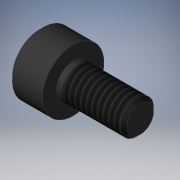
# Autodesk Inventor part: E-GSCB3-6
Saved by Autodesk Inventor 2019 (Build 230136000, 136)
## iProperties
Created: 2024-02-19
Part Number: E-GSCB3-6
Material: Generic
Catalog Web Link: www.cadenas.de
Description: E-GSCB-Economy Hexagon Socket Head Cap Screws - Stainless Steel
Vendor: MISUMI
Document SubType Name: Modeling
Designer: psAdmin
Manufacturer: MISUMI
Mass: 0.103858 g
Surface Area: 1.64097 cm^2
Volume: 0.103858 cm^3
Density: 1 g/cm^3
Appearance: PSOLRGB-175-175-175
Category: PARTsolutions
Company: MISUMI
Title: E-GSCB3-6
Author: Cadenas PARTsolutions
Comments: Economy Hexagon Socket Head Cap Screws - Stainless Steel
PSOL_IDENT_0: {$CADENAS_DATA/23d-libs/misumi/metric/27_screws_nuts/e_gscb.prj},160 {VTYP=3D},{NB=E-GSCB3-6},{LINA=
PSOL_IDENT_1: E-GSCB3-6},{NN=E-GSCB},{DATE=20.09.2023 07:17:35},{GEOMDATE=14.09.2023 02:41:30},{VERSION=},{LINEID=
PSOL_IDENT_2: 60},{WBVAR=L},{WBNUMERIC=L}  {NB=E-GSCB3-6},{LINA=E-GSCB3-6},{KT=DUMMY},{PN=E-GSCB3-6},{TYPE=E-GSCB}
PSOL_IDENT_3: ,{MAT=304 Stainless Steel Equivalent},{SC=A2-70},{M=3},{L=6},{L0=6,8,10,12,14,15,16,18,20,25,30},{LL=
PSOL_IDENT_4: Full Thread},{L1=18},{M1=3.0},{MP=3x0.5},{P=0.5},{A=5.5},{E=3},{B=2.5},{V=0.30}
NB: E-GSCB3-6
NN: E-GSCB
NT: Economy Hexagon Socket Head Cap Screws - Stainless Steel
NBSYN: $PN.
LINA: E-GSCB3-6
CATALOG: Misumi
PN: E-GSCB3-6
SC: A2-70
M: 3
L: 6
LL: Full Thread
MP: 3x0.5
A: 5.5
E: 3
B: 2.5
SUPPLIER: MISUMI
ARTICLENO: E-GSCB3-6
BOMINFO: E-GSCB3-6
CREATOR: CADENAS GmbH
Autodesk Inventor part; units mm, degrees
sketch "Sketch_1" plane through (0, 0, 0) normal (0, 0, 1) x (1, 0, 0)
  line L0 (6, 0) -> (-3, 0)
  line L1 (-3, 0) -> (-3, 2.45)
  line L2 (-3, 2.45) -> (-2.7, 2.75)
  line L3 (-2.7, 2.75) -> (0, 2.75)
  line L4 (0, 2.75) -> (0, 1.5)
  line L5 (0, 1.5) -> (5.6935, 1.5)
  line L6 (5.6935, 1.5) -> (6, 1.1935)
  line L7 (6, 1.1935) -> (6, 0)
  line L8 (6, 0) -> (-3, 0)
  constraints: 18 end point
revolve "Revolution1" add sketch "Sketch_1" angle 360 about axis through (6, 0, 0) along (1, 0, 0)
thread "Thread1" size "M3x0.5" class "6g" standard "ISO Metric profile" length 5.1935
sketch "Sketch2" plane through (-3, 0, 0) normal (-1, 0, 0) x (0, 0, 1)
  point P0 (0, 0)
hole "Hole1" at (-3, 0, 0) direction (1, 0, 0) diameter 2.5 depth 1.5 tip angle 150
sketch "Sketch_3" plane through (-3, 0, 0) normal (1, 0, 0) x (0, 0, -1)
  line L0 (-1.25, -0.7217) -> (0, -1.4434)
  line L1 (0, -1.4434) -> (1.25, -0.7217)
  line L2 (1.25, -0.7217) -> (1.25, 0.7217)
  line L3 (1.25, 0.7217) -> (0, 1.4434)
  line L4 (0, 1.4434) -> (-1.25, 0.7217)
  line L5 (-1.25, 0.7217) -> (-1.25, -0.7217)
  constraints: 12 end point
extrude "Extrusion1" cut sketch "Sketch_3" along normal blind 1.5
ref_plane "bolt_XY" through (0, 0, 0) normal (1, 0, 0) x (0, 0, -1)
ref_plane "bolt_YZ" through (0, 0, 0) normal (0, 0, -1) x (0, 1, 0)
ref_plane "bolt_ZX" through (0, 0, 0) normal (0, 1, 0) x (1, 0, 0)
ref_plane "nut_XY" through (6, 0, 0) normal (1, 0, 0) x (0, 0, -1)
ref_plane "nut_YZ" through (6, 0, 0) normal (0, 0, -1) x (0, 1, 0)
ref_plane "nut_ZX" through (6, 0, 0) normal (0, 1, 0) x (1, 0, 0)
body "Solid1"
